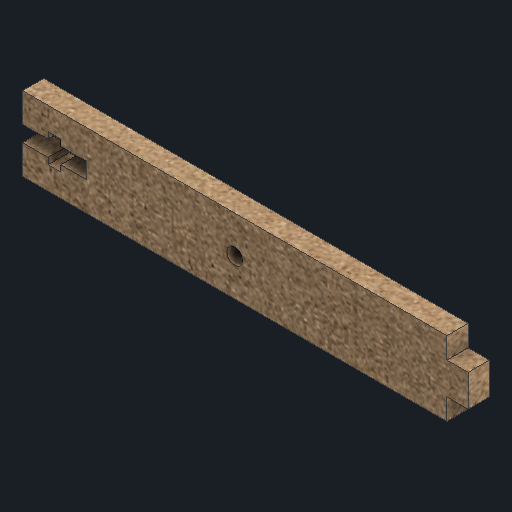
# Autodesk Inventor part: Magnet_Holder
Saved by Autodesk Inventor 2024.1 (Build 281209000, 209)
## iProperties
Created: 2023-08-05
Part Number: Magnet_Holder
Material: MDF Medium Density Fiberboard
Document SubType Name: Modeling
Designer: jaege
Density: 0.8 g/cm^3
Appearance: Cardboard - Corrugated
Author: jaege
Autodesk Inventor part; units mm, degrees
ref_plane "YZ Plane" through (0, 0, 0) normal (1, 0, 0) x (0, 1, 0)
ref_plane "XZ Plane" through (0, 0, 0) normal (0, 1, 0) x (-1, 0, 0)
ref_plane "XY Plane" through (0, 0, 0) normal (0, 0, 1) x (1, 0, 0)
sketch "Sketch1" plane through (0, 0, 0) normal (0, 0, 1) x (1, 0, 0)
  line L0 (88, 0) -> (88, 6) projected
  line L1 (84, 0) -> (88, 0) projected
  line L2 (84, 6) -> (84, 0) construction
  line L3 (84, 6) -> (88, 6) projected
  line L4 (4, -4) -> (84, -4)
  line L5 (84, -4) -> (84, 0)
  line L6 (84, 10) -> (4, 10)
  line L7 (84, 0) -> (84, 6) construction
  line L8 (84, 6) -> (84, 10)
  line L9 (4, 10) -> (4, -4)
  line L10 (4, 109.6455) -> (4, -35.8545) construction
  line L11 (4, 4.5) -> (16, 4.5)
  line L12 (16, 4.5) -> (16, 1.5)
  line L13 (16, 1.5) -> (4, 1.5)
  line L14 (4, 1.5) -> (4, 4.5)
  line L15 (8.8, 5.7) -> (11.2, 5.7)
  line L16 (11.2, 5.7) -> (11.2, 0.3)
  line L17 (11.2, 0.3) -> (8.8, 0.3)
  line L18 (8.8, 0.3) -> (8.8, 5.7)
  circle A0 centre (44, 3) radius 1.5
  line L19 (4, 10) -> (84, -4) construction
  point P0 (10, 5.7)
  point P1 (10, 4.5)
  point P2 (11.2, 3)
  point P3 (16, 3)
  point P4 (4, 3)
  point P5 (88, 3)
  point P6 (8.8, 4.5)
  point P7 (11.2, 4.5)
  point P8 (11.2, 1.5)
  point P9 (8.8, 1.5)
  dimension "d4" = 4
  dimension "d5" = 4
  dimension "d6" = 12
  dimension "d7" = 3
  dimension "d8" = 2.4
  dimension "d9" = 5.4
  dimension "d10" = 3
  constraints: 32 end point, 7 midpoint, 5 parallel, 5 perpendicular, 3 horizontal, 3 horizontal alignment, 3 vertical alignment, 1 centre point, 1 point on line, 1 vertical
  measures "d4" distance of L2.start L6.start
  measures "d5" distance of L4.end L1.start
  measures "d6" distance of L12.end L13.end
  measures "d7" distance of L11.end L12.end
  measures "d8" distance of L16.end L17.end
  measures "d9" distance of L15.end L16.end
  measures "d10" diameter of A0
extrude "Extrusion1" add sketch "Sketch1" along normal blind 4 contours L1 L5 L4 L9 L13 L18 L17 L16 L12 L11 L15 L6 L8 L3 L0
body "Solid1"
